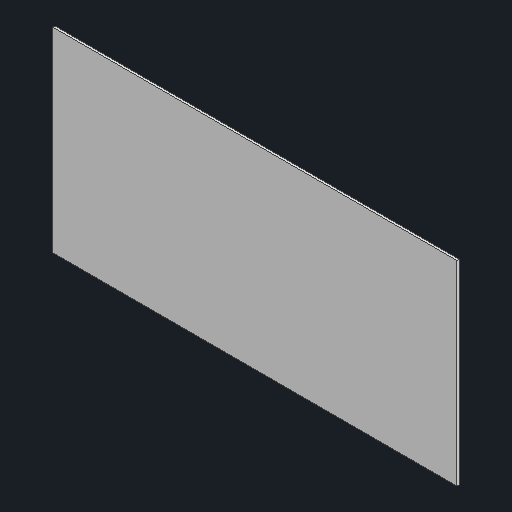
# Autodesk Inventor part: стенка ответная
Saved by Autodesk Inventor 2025 (Build 290162000, 162)
## iProperties
Created: 2025-10-03
Part Number: стенка ответная
Material: Типовые
Document SubType Name: Modeling
Designer: Phantom
Density: 1 g/cm^3
Appearance: По умолчанию
Author: Phantom
Autodesk Inventor part; units mm, degrees
ref_plane "YZ Plane" through (0, 0, 0) normal (1, 0, 0) x (0, 1, 0)
ref_plane "XZ Plane" through (0, 0, 0) normal (0, 1, 0) x (-1, 0, 0)
ref_plane "XY Plane" through (0, 0, 0) normal (0, 0, 1) x (1, 0, 0)
sketch "Эскиз1" plane through (0, 0, 0) normal (0, 0, 1) x (1, 0, 0)
  line L0 (0, 0) -> (380, 0)
  line L1 (380, 0) -> (380, 227)
  line L2 (380, 227) -> (0, 227)
  line L3 (0, 227) -> (0, 0)
  dimension "d0" = 380
  dimension "d1" = 227
  constraints: 8 end point, 2 parallel, 1 horizontal, 1 perpendicular
  measures "d0" distance of L2.end L1.end
  measures "d1" distance of L1.end L0.end
extrude "Выдавливание1" add sketch "Эскиз1" along normal blind 2
sketch "Эскиз2" plane through (0, 0, 2) normal (0, 0, 1) x (1, 0, 0)
  arc A0 (24, 227) -> (184.1593, 0) centre (184.1593, 170) ccw projected
  line L0 (380, 0) -> (380, 227) projected
  line L1 (380, 227) -> (0, 227) projected
  line L2 (0, 227) -> (0, 0) projected
  line L3 (0, 0) -> (380, 0) projected
  line L4 (14.1593, 232.9564) -> (14.1593, -21.9054)
  line L5 (0, 227) -> (0, 0) projected
  point P0 (14.1593, 170)
  point P1 (24, 227)
  point P2 (14.1593, 0)
  constraints: 2 end point, 1 parallel, 1 tangent
extrude "Выдавливание2" cut sketch "Эскиз2" against normal blind 10 contours A0 L4 L1 | L4 L3 L2 L1
sketch "Эскиз3" plane through (0, 0, 0) normal (0, 0, -1) x (-1, 0, 0)
  circle A0 centre (-192.6104, 161.8048) radius 3.1 projected
  line L0 (-192.6104, 161.8048) -> (-192.6104, 176.8048)
  line L1 (-192.6104, 176.8048) -> (-426.6328, 176.8048)
  line L2 (-14.1593, 0) -> (-14.1593, 170) projected
  arc A1 (-14.1593, 170) -> (-24, 227) centre (-184.1593, 170) ccw projected
  line L3 (-380, 227) -> (-24, 227) projected
  line L4 (-380, 0) -> (-380, 227) projected
  line L5 (-14.1593, 0) -> (-380, 0) projected
  line L6 (-192.6104, 176.8048) -> (46.0253, 176.8048)
  point P0 (0, 0)
  point P1 (-380, 176.8048)
  point P2 (-14.2955, 176.8048)
  dimension "d6" = 15
  constraints: 6 end point, 1 horizontal, 1 perpendicular, 1 vertical
  measures "d6" distance of L0.start L0.end
extrude "Выдавливание3" cut sketch "Эскиз3" against normal blind 10 contours L1 L4 L3 A1 L6
